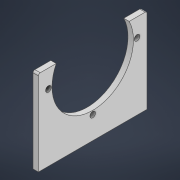
# Autodesk Inventor part: łapa1
Saved by Autodesk Inventor 2022 (Build 260153000, 153)
## iProperties
Created: 2023-04-12
Part Number: łapa1
Material: Ogólny
Document SubType Name: Modeling
Designer: jacek
Density: 1 g/cm^3
Appearance: Domyślna
Author: jacek
Autodesk Inventor part; units mm, degrees
ref_plane "YZ Plane" through (0, 0, 0) normal (1, 0, 0) x (0, 1, 0)
ref_plane "XZ Plane" through (0, 0, 0) normal (0, 1, 0) x (-1, 0, 0)
ref_plane "XY Plane" through (0, 0, 0) normal (0, 0, 1) x (1, 0, 0)
sketch "Szkic1" plane through (0, 0, 0) normal (1, 0, 0) x (0, 1, 0)
  line L0 (0, 0) -> (6, 0)
  line L1 (6, 0) -> (6, -178)
  line L2 (6, -178) -> (0, -178)
  line L3 (0, -178) -> (0, 0)
  line L4 (0, -89) -> (100, -89)
  line L5 (100, -129.3113) -> (100, -149)
  line L6 (100, -149) -> (6, -149)
  line L7 (100, -48.6887) -> (100, -29)
  line L8 (100, -29) -> (6, -29)
  line L9 (100, -89) -> (80, -89)
  arc A0 (100, -48.6887) -> (100, -129.3113) centre (80, -89) ccw
  line L10 (80, -40) -> (80, -138)
  point P0 (6, -29)
  dimension "d0" = 6
  dimension "d1" = 178
  dimension "d2" = 100
  dimension "d3" = 60
  dimension "d4" = 20
  dimension "d5" = 90
  dimension "d6" = 98
  constraints: 22 end point, 2 horizontal, 2 midpoint, 2 parallel, 2 perpendicular, 2 point on circle, 2 point on line, 2 symmetric about line, 2 vertical, 1 centre point, 1 coincident
  measures "d0" distance of L1.end L2.end
  measures "d1" distance of L0.end L1.end
  measures "d2" distance of L4.start L4.end
  measures "d3" distance of L4.end L5.end
  measures "d4" distance of L9.end L4.end
  measures "d5" diameter of A0
  measures "d6" distance of L10.start L10.end
extrude "Wyciągnięcie proste1" add sketch "Szkic1" against normal blind 6 contours L0 L1 L4 L3 | L4 L1 L2 L3 | L8 L7 A0 L4 L1 | L4 A0 L5 L6 L1
hole "Otwór1" at (0, 80, -40) at (0, 80, -138) direction (-1, 0, 0) diameter 6.2 depth 33 tip angle 118
pattern_circular "Szyk kołowy1" count 4 over 360 about axis through (0, 80, -89) along (-1, 0, 0) of "Otwór1"
fillet "Zaokrąglenie1" radius 2 2 edges at (-3, 100, -29) (-3, 100, -149)
extrude "Wyciągnięcie proste3" cut sketch "Szkic1" against normal blind 37.25 contours L0 L1 L4 L3 | L4 L1 L2 L3
